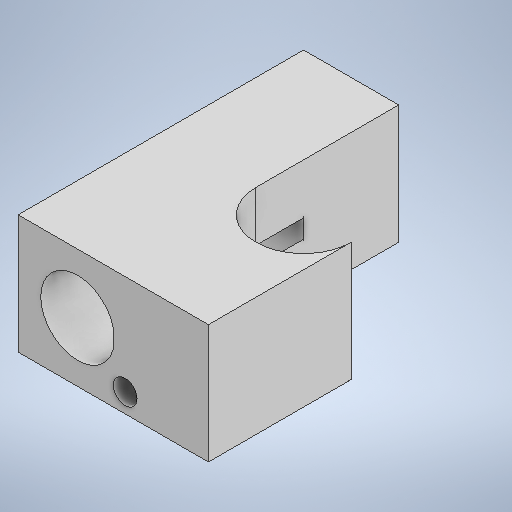
# Autodesk Inventor part: rod4.5
Saved by Autodesk Inventor 2025 (Build 290162000, 162)
## iProperties
Created: 2024-07-14
Part Number: rod4.5
Material: 一般
Document SubType Name: Modeling
Designer: Saigusa
Density: 1 g/cm^3
Appearance: 既定
Author: Saigusa
Autodesk Inventor part; units mm, degrees
ref_plane "YZ Plane" through (0, 0, 0) normal (1, 0, 0) x (0, 1, 0)
ref_plane "XZ Plane" through (0, 0, 0) normal (0, 1, 0) x (-1, 0, 0)
ref_plane "XY Plane" through (0, 0, 0) normal (0, 0, 1) x (1, 0, 0)
sketch "スケッチ1" plane through (0, 0, 0) normal (0, 1, 0) x (-1, 0, 0)
  circle A0 centre (0, 0) radius 1.15
  circle A1 centre (0, 0) radius 2
  line L0 (0, 0) -> (6, 0)
  line L1 (6, 0) -> (6, 6)
  line L2 (6, 6) -> (0, 6)
  line L3 (0, 6) -> (0, 0)
  line L4 (0, 0) -> (6, 0)
  line L5 (6, 0) -> (6, -6)
  line L6 (6, -6) -> (0, -6)
  line L7 (0, -6) -> (0, 0)
  line L8 (0, 2) -> (2, 2)
  line L9 (2, 2) -> (2, -6)
  line L10 (2, -6) -> (0, -6)
  line L11 (0, -6) -> (0, 2)
  line L12 (0, 6) -> (-2, 6)
  line L13 (-2, 6) -> (-2, 0)
  line L14 (-2, 0) -> (0, 0)
  line L15 (0, 0) -> (0, 6)
  point P0 (2, 0)
  dimension "d0" = 2.3
  dimension "d1" = 4
  dimension "d2" = 6
  dimension "d3" = 6
  dimension "d4" = 6
  constraints: 32 end point, 8 parallel, 4 horizontal, 4 perpendicular, 4 point on line, 2 centre point, 2 coincident, 2 point on circle
  measures "d0" diameter of A0
  measures "d1" diameter of A1
  measures "d2" distance of L2.end L1.end
  measures "d3" distance of L1.end L0.end
  measures "d4" distance of L4.end L5.end
extrude "押し出し1" add sketch "スケッチ1" along normal blind 5 contours L9 L8 L3 L2 L1 L0 | A1 L8 L9 | L0 L5 L6 L9 | A1 L13 L12 L3
sketch "スケッチ2" plane through (-6, 0, 6) normal (0, 0, 1) x (1, 0, 0)
  line L0 (0, 0) -> (8, 0) projected
  line L1 (0, 5) -> (8, 5) projected
  line L2 (8, 0) -> (4, 0)
  line L3 (4, 0) -> (4, 5)
  line L4 (4, 5) -> (8, 5)
  line L5 (8, 5) -> (8, 0)
  line L6 (4, 0) -> (4.5, 0)
  line L7 (4.5, 0) -> (4.5, 0.8)
  line L8 (4.5, 0.8) -> (4, 0.8)
  line L9 (4, 0.8) -> (4, 0)
  circle A0 centre (4.5, 0.8) radius 0.5
  line L10 (0, 5) -> (2.5, 5)
  line L11 (2.5, 5) -> (2.5, 2.5)
  line L12 (2.5, 2.5) -> (0, 2.5)
  line L13 (0, 2.5) -> (0, 5)
  circle A1 centre (2.5, 2.5) radius 1.55
  point P0 (6, 0)
  point P1 (4, 2.8905)
  point P2 (4, 2.1095)
  dimension "d7" = 4
  dimension "d8" = 0.5
  dimension "d9" = 0.8
  dimension "d10" = 2.5
  dimension "d11" = 2.5
  dimension "d12" = 3.1
  constraints: 24 end point, 6 parallel, 3 horizontal, 3 perpendicular, 2 coincident, 1 centre point, 1 horizontal alignment, 1 midpoint, 2 other
  measures "d7" distance of L3.end L4.end
  measures "d8" distance of L8.end L7.end
  measures "d9" distance of L7.end L6.end
  measures "d10" distance of L11.end L12.end
  measures "d11" distance of L10.end L11.end
  measures "d12" diameter of A1
extrude "押し出し2" cut sketch "スケッチ2" against normal blind 8 contours A0 L7 L8 | L8 L7 A0 | A1 L12 L11 L3 | A1 L11 L12
